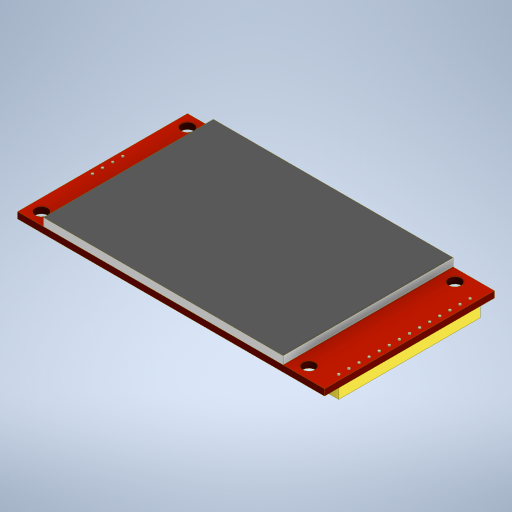
# Autodesk Inventor part: LCD9341
Saved by Autodesk Inventor 2024 (Build 280153000, 153)
## iProperties
Created: 2023-10-07
Part Number: LCD9341
Material: Generic
Document SubType Name: Modeling
Designer: chris
Density: 1 g/cm^3
Appearance: Default(5)
Author: chris
Autodesk Inventor part; units mm, degrees
ref_plane "YZ Plane" through (0, 0, 0) normal (1, 0, 0) x (0, 1, 0)
ref_plane "XZ Plane" through (0, 0, 0) normal (0, 1, 0) x (-1, 0, 0)
ref_plane "XY Plane" through (0, 0, 0) normal (0, 0, 1) x (1, 0, 0)
sketch "Sketch1" plane through (0, 0, 0) normal (0, 1, 0) x (-1, 0, 0)
  line L0 (-38.59, 21.36) -> (38.59, 21.36)
  line L1 (38.59, 21.36) -> (38.59, -21.36)
  line L2 (38.59, -21.36) -> (-38.59, -21.36)
  line L3 (-38.59, -21.36) -> (-38.59, 21.36)
  line L4 (-38.59, 21.36) -> (38.59, -21.36) construction
  line L5 (38.59, 21.36) -> (-38.59, -21.36) construction
  point P0 (0, 0)
  dimension "d0" = 42.72
  dimension "d1" = 77.18
  constraints: 12 end point, 2 midpoint, 2 parallel, 1 horizontal, 1 perpendicular
  measures "d0" distance of L0.end L1.end
  measures "d1" distance of L1.end L2.end
extrude "Extrusion1" add sketch "Sketch1" along normal blind 1.6
sketch "Sketch2" plane through (0, 1.6, 0) normal (0, 1, 0) x (1, 0, 0)
  line L0 (38.59, 21.36) -> (-38.59, 21.36) projected
  line L1 (28.18, -21.36) -> (-32.08, -21.36)
  line L2 (-32.08, -21.36) -> (-32.08, 21.36)
  line L3 (-32.08, 21.36) -> (28.18, 21.36)
  line L4 (28.18, 21.36) -> (28.18, -21.36)
  line L5 (28.18, -21.36) -> (-32.08, 21.36) construction
  line L6 (-32.08, -21.36) -> (28.18, 21.36) construction
  line L7 (38.59, -21.36) -> (38.59, 21.36) projected
  line L8 (-38.59, 21.36) -> (-38.59, -21.36) projected
  dimension "d4" = 60.26
  dimension "d5" = 10.41
  constraints: 12 end point, 3 parallel, 1 horizontal, 1 perpendicular, 1 point on line
  measures "d4" distance between parallel lines of L4 L2
  measures "d5" distance between parallel lines of L7 L4
extrude "Extrusion2" add sketch "Sketch2" along normal blind 2 separate body
sketch "Sketch3" plane through (0, 1.6, 0) normal (0, 1, 0) x (1, 0, 0)
  line L0 (38.59, -21.36) -> (38.59, 21.36) projected
  line L1 (38.59, 21.36) -> (-38.59, 21.36) projected
  line L2 (-38.59, -21.36) -> (38.59, -21.36) projected
  line L3 (-38.59, 21.36) -> (-38.59, -21.36) projected
  point P0 (0, 0)
  point P1 (31.67, 18.36)
  point P2 (28.18, 21.36)
  point P3 (31.67, -18.36)
  point P4 (-35.59, -18.36)
  point P5 (-35.59, 18.36)
  point P6 (-32.08, -21.36)
  dimension "d8" = 6.92
  dimension "d9" = 3
  dimension "d11" = 3
  dimension "d12" = 3
  constraints: 2 horizontal alignment, 2 vertical alignment
  measures "d8" distance from line of L0 point (31.67, 18.36)
  measures "d9" distance from line of L1 point (31.67, 18.36)
  measures "d11" distance from line of L3 point (-35.59, 18.36)
  measures "d12" distance from line of L2 point (-35.59, -18.36)
hole "Hole1" at (31.67, 1.6, -18.36) at (31.67, 1.6, 18.36) at (-35.59, 1.6, 18.36) at (-35.59, 1.6, -18.36) direction (0, -1, 0) diameter 3.2 end through all bodies 1
sketch "Sketch4" plane through (0, 0, 0) normal (0, -1, 0) x (1, 0, 0)
  line L0 (36.05, 17.78) -> (38.59, 17.78)
  line L1 (38.59, 17.78) -> (38.59, -17.78)
  line L2 (38.59, -17.78) -> (36.05, -17.78)
  line L3 (36.05, -17.78) -> (36.05, 17.78)
  line L4 (38.59, 21.36) -> (38.59, -21.36) projected
  line L5 (38.59, -21.36) -> (-38.59, -21.36) projected
  line L6 (-38.59, -5.08) -> (-36.05, -5.08)
  line L7 (-36.05, -5.08) -> (-36.05, 5.08)
  line L8 (-36.05, 5.08) -> (-38.59, 5.08)
  line L9 (-38.59, 5.08) -> (-38.59, -5.08)
  line L10 (-38.59, -21.36) -> (-38.59, 21.36) projected
  point P0 (0, 0)
  point P1 (37.32, -16.51)
  dimension "d20" = 2.54
  dimension "d21" = 1.27
  dimension "d22" = 1.27
  dimension "d23" = 4.85
  dimension "d24" = 35.56
  dimension "d39" = 2.54
  dimension "d40" = 10.16
  dimension "d41" = 5.08
  constraints: 16 end point, 4 parallel, 2 collinear, 2 horizontal, 2 perpendicular
  measures "d20" distance between parallel lines of L3 L1
  measures "d21" distance from line of L3 point (37.32, -16.51)
  measures "d22" distance from line of L2 point (37.32, -16.51)
  measures "d23" distance from line of L5 point (37.32, -16.51)
  measures "d24" distance between parallel lines of L0 L2
  measures "d39" distance of L7.end L8.end
  measures "d40" distance of L6.end L7.end
  measures "d41" distance from line of point (0, 0) L8
extrude "Extrusion3" add sketch "Sketch4" along normal blind 2.5 separate body
sketch "Sketch5" plane through (0, 1.6, 0) normal (0, 1, 0) x (1, 0, 0)
  line L0 (38.59, 21.36) -> (-38.59, 21.36) projected
  line L1 (38.59, -21.36) -> (38.59, 21.36) projected
  circle A0 centre (37.32, 16.51) radius 0.3
  circle A1 centre (37.32, 13.97) radius 0.3
  circle A2 centre (37.32, 11.43) radius 0.3
  circle A3 centre (37.32, 8.89) radius 0.3
  circle A4 centre (37.32, 6.35) radius 0.3
  circle A5 centre (37.32, 3.81) radius 0.3
  circle A6 centre (37.32, 1.27) radius 0.3
  circle A7 centre (37.32, -1.27) radius 0.3
  circle A8 centre (37.32, -3.81) radius 0.3
  circle A9 centre (37.32, -6.35) radius 0.3
  circle A10 centre (37.32, -8.89) radius 0.3
  circle A11 centre (37.32, -11.43) radius 0.3
  circle A12 centre (37.32, -13.97) radius 0.3
  circle A13 centre (37.32, -16.51) radius 0.3
  line L2 (-38.59, 21.36) -> (-38.59, -21.36) projected
  circle A14 centre (-37.32, 3.81) radius 0.3
  circle A15 centre (-37.32, 1.27) radius 0.3
  circle A16 centre (-37.32, -1.27) radius 0.3
  circle A17 centre (-37.32, -3.81) radius 0.3
  point P0 (0, 0)
  dimension "d27" = 4.85
  dimension "d28" = 1.27
  dimension "d29" = 0.6
  dimension "d32" = 2.54
  dimension "d42" = 1.27
  dimension "d43" = 3.81
  dimension "d47" = 2.54
  constraints: 18 centre point, 18 coincident, 2 vertical, 1 equal radius, 48 other
  measures "d27" distance from line of L0 point (37.32, 16.51)
  measures "d28" distance from line of L1 point (37.32, 16.51)
  measures "d29" diameter of A0
  measures "d32" distance of A0.centre A1.centre
  measures "d42" distance from line of L2 point (-37.32, 3.81)
  measures "d43" vertical distance of point (-37.32, 3.81) point (0, 0)
  measures "d47" distance of A14.centre A15.centre
extrude "Extrusion4" add sketch "Sketch5" along normal blind 0.2 separate body
body "Solid1"
body "Solid2"
body "Solid3"
body "Solid4"
